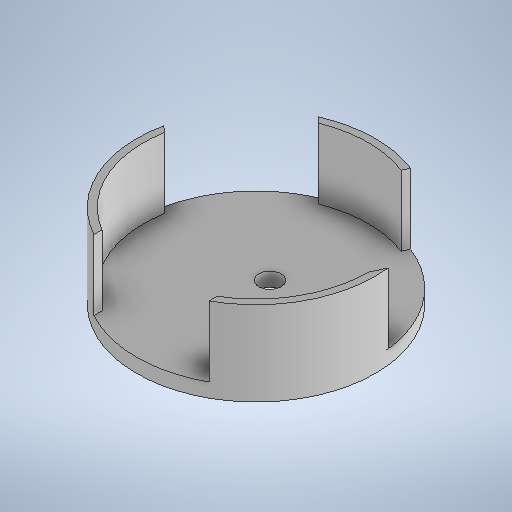
# Autodesk Inventor part: Part4
Saved by Autodesk Inventor 2025.4 (Build 294407000, 407)
## iProperties
Created: 2026-03-03
Part Number: Part4
Material: Generic
Document SubType Name: Modeling
Designer: Amir
Density: 1 g/cm^3
Appearance: Default
Author: Amir
Autodesk Inventor part; units mm, degrees
ref_plane "YZ Plane" through (0, 0, 0) normal (1, 0, 0) x (0, 1, 0)
ref_plane "XZ Plane" through (0, 0, 0) normal (0, 1, 0) x (-1, 0, 0)
ref_plane "XY Plane" through (0, 0, 0) normal (0, 0, 1) x (1, 0, 0)
sketch "Sketch1" plane through (0, 0, 0) normal (0, 0, 1) x (1, 0, 0)
  line L0 (17.5, 11.2702) -> (17.5, 14.0313)
  line L1 (-17.5, 14.0313) -> (-17.5, 11.2702)
  line L2 (20.5, 12.771) -> (20.5, 15.6525)
  line L3 (-20.5, 15.6525) -> (-20.5, 12.771)
  arc A0 (17.5, 14.0313) -> (-17.5, 14.0313) centre (0, 50) ccw
  line L4 (40, 50.029) -> (42.2274, 54.8057)
  line L5 (39.7713, 54.271) -> (41.6722, 58.3474)
  circle A1 centre (0, 50) radius 42.5
  arc A2 (-41.0627, 60.9592) -> (-38.9529, 59.0922) centre (1.7976, 107.2672) ccw
  arc A3 (-18.7749, 88.1281) -> (-16.8719, 86.2676) centre (1.7976, 107.2672) ccw
  arc A4 (-16.8563, 89.0143) -> (-14.8286, 87.1499) centre (1.7976, 107.2672) ccw
  line L6 (16.2129, 86.5669) -> (17.2697, 88.8331)
  line L7 (14.3631, 87.3323) -> (15.422, 89.6032)
  arc A5 (-41.5922, 58.7372) -> (-39.406, 56.8678) centre (1.7976, 107.2672) ccw
  circle A6 centre (0, 55) radius 4
  line L8 (-6, 53.75) -> (6, 53.75)
  line L9 (6, 53.75) -> (6, 56.25)
  line L10 (6, 56.25) -> (-6, 56.25)
  line L11 (-6, 56.25) -> (-6, 53.75)
  point P0 (0, 0)
  point P1 (20.5, 12.771)
  point P2 (42.2274, 54.8057)
  point P3 (-17.5, 11.2702)
  point P4 (17.5, 11.2702)
  point P5 (41.6722, 58.3474)
  point P6 (15.422, 89.6032)
  point P7 (17.2697, 88.8331)
  point P8 (-18.7749, 88.1281)
  point P9 (-16.8563, 89.0143)
  point P10 (-41.0627, 60.9592)
  point P11 (-3.7997, 53.75)
  point P12 (3.7997, 53.75)
  point P13 (3.7997, 56.25)
  point P14 (-3.7997, 56.25)
  point P15 (0, 44.1942)
  dimension "d87" = 40
  dimension "d167" = 85
  dimension "d168" = 2.5
  dimension "d33" = 2
  dimension "d79" = 3
  dimension "d80" = 3
  dimension "d81" = 35
  dimension "d92" = 2
  dimension "d93" = 35
  dimension "d94" = 50
  dimension "d95" = 17.5
  dimension "d146" = 8
  dimension "d147" = 12
  dimension "d148" = 2.5
  dimension "d153" = 55
  dimension "d154" = 1.25
  dimension "d169" = 35
  constraints: 24 end point, 8 point on circle, 6 parallel, 5 centre point, 1 coincident, 1 horizontal, 1 perpendicular, 1 vertical alignment, 28 other
  measures "d33" distance between parallel lines of L4 L5
  measures "d79" distance between parallel lines of L1 L3
  measures "d80" distance between parallel lines of L2 L0
  measures "d81" distance between parallel lines of L1 L0
  measures "d92" distance between parallel lines of L6 L7
  measures "d93" distance between parallel lines of L5 L6
  measures "d94" distance of point (0, 50) point (0, 0)
  measures "d95" distance from line of L0 point (0, 0)
  measures "d146" diameter of A6
  measures "d147" distance of L10.end L9.end
  measures "d148" distance of L9.end L8.end
  measures "d153" distance of point (0, 0) A6.centre
  measures "d154" distance from line of A6.centre L8
  measures "d169" radial gap between concentric circles of A2 A3
extrude "Extrusion12" add sketch "Sketch1" along normal blind 5 contours A1 L1 A0 L0 | L0 A0 L2 A1 | A1 L3 A0 L1 | L2 A0 L4 A1 | A1 A5 A0 L3 | A0 L5 A1 L4 | A1 A2 A0 A5 | A0 L6 A1 L5 | A1 A3 A0 A2 | A0 L7 A1 L6 | A1 A4 A0 A3 | A0 A4 A1 L7 | A6 L8 L10 | A6 L10 L9 L8 | L10 A6 | A6 L8 | A6 L8 L11 L10
extrude "Extrusion13" add sketch "Sketch1" along normal blind 5 contours A1 L1 A0 L0 | A6 L8 L10 | A6 L10 L9 L8 | L10 A6 | A6 L8 | A6 L8 L11 L10
extrude "Extrusion14" cut sketch "Sketch1" along normal blind 17 contours A6 L8 L10 | A6 L10 L9 L8 | L10 A6 | A6 L8 | A6 L8 L11 L10
extrude "Extrusion15" add sketch "Sketch1" along normal blind 5 contours A6 L10 L9 L8 | A6 L8 L11 L10
extrude "Extrusion16" add sketch "Sketch1" along normal blind 30 contours L2 A0 L4 A1 | A1 A5 A0 L3 | A0 L7 A1 L6 | A0 A4 A1 L7
extrude "Extrusion17" add sketch "Sketch1" along normal blind 30 contours L0 A0 L2 A1 | A1 L3 A0 L1 | A0 L5 A1 L4 | A1 A2 A0 A5 | A1 A4 A0 A3
extrude "Extrusion18" cut sketch "Sketch1" along normal blind 30 contours L0 A0 L2 A1 | A1 L3 A0 L1 | A0 L5 A1 L4 | A1 A2 A0 A5 | A0 L7 A1 L6 | A1 A4 A0 A3
extrude "Extrusion19" add sketch "Sketch1" along normal blind 5 contours L0 A0 L2 A1 | A1 L3 A0 L1 | A0 L5 A1 L4 | A1 A2 A0 A5 | A0 L7 A1 L6 | A1 A4 A0 A3
body "Solid2"
